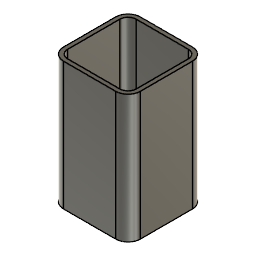
▢-60×60×3.2 (Autodesk Fusion 360 design; units mm, degrees)
Autodesk Fusion 360 part; units mm, degrees
sketch "スケッチ1" plane through (0, 0, 0) normal (0, 0, 1) x (1, 0, 0)
  arc A0 (61.3889, -110.2463) -> (70.9889, -100.6463) centre (61.3889, -100.6463) ccw
  arc A1 (61.3889, -107.0463) -> (67.7889, -100.6463) centre (61.3889, -100.6463) ccw
  arc A2 (70.9889, -59.8463) -> (61.3889, -50.2463) centre (61.3889, -59.8463) ccw
  arc A3 (67.7889, -59.8463) -> (61.3889, -53.4463) centre (61.3889, -59.8463) ccw
  arc A4 (20.5889, -50.2463) -> (10.9889, -59.8463) centre (20.5889, -59.8463) ccw
  arc A5 (20.5889, -53.4463) -> (14.1889, -59.8463) centre (20.5889, -59.8463) ccw
  line L0 (20.5889, -110.2463) -> (61.3889, -110.2463)
  line L1 (20.5889, -107.0463) -> (61.3889, -107.0463)
  line L2 (10.9889, -59.8463) -> (10.9889, -100.6463)
  line L3 (14.1889, -59.8463) -> (14.1889, -100.6463)
  arc A6 (10.9889, -100.6463) -> (20.5889, -110.2463) centre (20.5889, -100.6463) ccw
  arc A7 (14.1889, -100.6463) -> (20.5889, -107.0463) centre (20.5889, -100.6463) ccw
  line L4 (61.3889, -50.2463) -> (20.5889, -50.2463)
  line L5 (61.3889, -53.4463) -> (20.5889, -53.4463)
  line L6 (70.9889, -100.6463) -> (70.9889, -59.8463)
  line L7 (67.7889, -100.6463) -> (67.7889, -59.8463)
  point P0 (40.9889, -80.2463)
extrude "押し出し1" add sketch "スケッチ1" along normal blind 100
